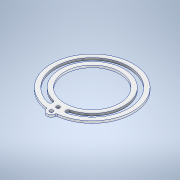
# Autodesk Inventor part: lock ring 2
Saved by Autodesk Inventor 2021 (Build 250183000, 183)
## iProperties
Created: 2021-03-30
Part Number: lock ring 2
Material: Aluminum 6061
Document SubType Name: Modeling
Designer: Work
Density: 2.7 g/cm^3
Appearance: Aluminum - Flat
Mass: 34.3249 g
Surface Area: 118.816 cm^2
Volume: 12.7129 cm^3
Author: Work
Autodesk Inventor part; units mm, degrees
ref_plane "YZ Plane" through (0, 0, 0) normal (1, 0, 0) x (0, 1, 0)
ref_plane "XZ Plane" through (0, 0, 0) normal (0, 1, 0) x (-1, 0, 0)
ref_plane "XY Plane" through (0, 0, 0) normal (0, 0, 1) x (1, 0, 0)
sketch "Sketch1" plane through (0, 0, 0) normal (0, 1, 0) x (-1, 0, 0)
  arc A0 (-9.3914, 47.3099) -> (9.3914, 47.3099) centre (0, 0) ccw
  arc A1 (-11.6619, 43.5227) -> (11.6619, 43.5227) centre (0, 0) ccw
  arc A2 (-13.3054, 49.6564) -> (13.3054, 49.6564) centre (0, 0) ccw
  circle A3 centre (0, 0) radius 38.708
  circle A4 centre (12.4836, 46.5895) radius 3.175
  circle A5 centre (-12.4836, 46.5895) radius 3.175
  line L0 (0, 0) -> (12.4836, 46.5895)
  line L1 (0, 0) -> (-12.4836, 46.5895)
  line L2 (0, 0) -> (0, 57.758)
  arc A6 (6.2927, 58.6092) -> (-6.2927, 58.6092) centre (0, 57.758) ccw
  arc A7 (6.2927, 58.6092) -> (7.6555, 57.2484) centre (7.8659, 58.8219) ccw
  arc A8 (-7.6555, 57.2484) -> (-6.2927, 58.6092) centre (-7.8659, 58.8219) ccw
  arc A9 (-7.6555, 57.2484) -> (7.6555, 57.2484) centre (0, 0) ccw
  point P0 (0, 48.233)
  point P1 (11.6619, 43.5227)
  point P2 (-11.6619, 43.5227)
  dimension "d0" = 96.4661
  dimension "d1" = 3.175
  dimension "d2" = 3.175
  dimension "d3" = 6.35
  dimension "d5" = 6.35
  dimension "d6" = 6.35
  dimension "d9" = 15
  dimension "d10" = 15
  dimension "d11" = 12.7
  dimension "d12" = 3.175
  dimension "d13" = 3.175
  dimension "d14" = 6.35
  dimension "d15" = 57.758
  dimension "d16" = 9.525
  constraints: 21 point on circle, 10 centre point, 6 end point, 4 tangent, 2 coincident, 2 point on line, 1 vertical
  measures "d0" diameter of A0
  measures "d1" radial gap between concentric circles of A0 A1
  measures "d2" radial gap between concentric circles of A0 A2
  measures "d3" radial gap between concentric circles of A1 A3
  measures "d5" diameter of A4
  measures "d6" diameter of A5
  measures "d9" angle of L2 L1
  measures "d10" angle of L2 L0
  measures "d11" diameter of A6
  measures "d12" diameter of A7
  measures "d13" diameter of A8
  measures "d14" radial gap between concentric circles of A9 A2
  measures "d15" distance of L0.start L2.end
  measures "d16" distance of point (0, 48.233) A6.centre
extrude "Extrusion1" add sketch "Sketch1" along normal blind 3.175 contours L1 A3 L0 A1 | A7 A9 A8 A6
hole "Hole1" at (0, 0, 48.233) at (0, 0, 57.758) direction (0, 1, 0) diameter 4.9784 end through all clearance for "Flat Head Machine Screw (82)" size "#10" standard "Ansi Unified Screw Threads"
equation "\"d0\" = ringDiam"
equation "\"d9\" = stageAngle"
equation "\"d10\" = stageAngle"
equation "\"d11\" = thickness"
equation "\"height\" = 203.2"
equation "\"thickness\" = 12.7"
equation "\"shaftDiam\" = 6.35"
equation "\"shaftSpace\" = 1.5875"
equation "\"stageSpace\" = 2.54"
equation "\"stageAngle\" = 15deg"
equation "\"bearingDiam\" = 9.5504"
equation "\"FlangeDiam\" = 12.7"
equation "\"FlangeDepth\" = 1.5875"
equation "\"smallFilet\" = 0.39687"
equation "\"ringDiam\" = 96.46608"
equation "\"stockHeight\" = 50.8"
equation "\"stockWidth\" = 76.2"
equation "\"stockRad\" = 9.525"
equation "\"stockGuage\" = 3.175"
equation "\"groundActu\" = 304.8"
equation "\"baseWidth\" = 1066.8"
equation "\"baseDepth\" = 254"
equation "\"capThickness\" = 3.175"
equation "\"sup1Len\" = 660.4"
equation "\"sup1Ang\" = 22.619865deg"
equation "\"sup2Len\" = 2079.37366"
equation "\"sup2Ang\" = 8.959949deg"
equation "\"supVertLen\" = 955.13561"
equation "\"supSideLen\" = 1531.12879"
equation "\"supSideAng\" = 19.376933deg"
body "Solid1"
